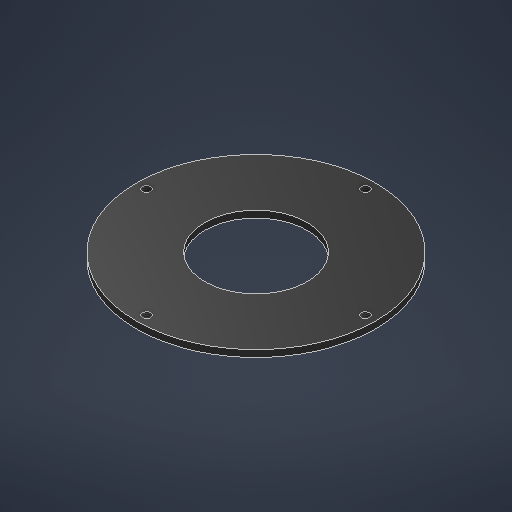
# Autodesk Inventor part: STRAIN_WAVE_BASS_PLATE,REV-ENG
Saved by Autodesk Inventor 2026.2 (Build 302298010, 298A)
## iProperties
Created: 2026-03-06
Part Number: STRAIN_WAVE_BASS_PLATE,REV-ENG
Material: Steel, 4140
Document SubType Name: Sheet Metal
Designer: 4aida
Density: 7.87 g/cm^3
Sheet Metal Rule: Default_mm
Appearance: Anodized - Dark Gray
Author: 4aida
Autodesk Inventor part; units mm, degrees
(part 1 of 3)
ref_plane "YZ Plane" through (0, 0, 0) normal (1, 0, 0) x (0, 1, 0)
ref_plane "XZ Plane" through (0, 0, 0) normal (0, 1, 0) x (-1, 0, 0)
ref_plane "XY Plane" through (0, 0, 0) normal (0, 0, 1) x (1, 0, 0)
sketch "Sketch1" plane through (0, 0, 0) normal (0, 1, 0) x (-1, 0, 0)
  circle A0 centre (0, 0) radius 15
  circle A1 centre (0, 0) radius 35
  dimension "d0" = 30
  dimension "d1" = 70
  measures "d0" diameter of A0
  measures "d1" diameter of A1
extrude "Plate1" add sketch "Sketch1" along normal blind 2
sketch "Sketch2" plane through (0, 0, 0) normal (0, -1, 0) x (1, 0, 0)
  line L0 (-32, -32) -> (32, -32)
  line L1 (32, -32) -> (32, 32)
  line L2 (32, 32) -> (-32, 32)
  line L3 (-32, 32) -> (-32, -32)
  line L4 (-32, -32) -> (32, 32) construction
  line L5 (32, -32) -> (-32, 32) construction
  point P0 (0, 0)
  point P1 (0, 32)
  point P2 (32, 0)
  point P3 (0, -32)
  point P4 (-32, 0)
  point P5 (32, 0)
  point P6 (0, -32)
  point P7 (-32, 0)
  point P8 (0, 32)
  dimension "d3" = 64
  constraints: 12 end point, 6 midpoint, 4 coincident, 2 parallel, 2 perpendicular, 1 horizontal
  measures "d3" distance between parallel lines of L3 L1
hole "Hole1" at (0, 0, 32) at (32, 0, 0) at (0, 0, -32) at (-32, 0, 0) direction (0, 1, 0) diameter 2.459 end through all thread size "M3x0.5" class "6H" standard "ANSI Metric M Profile"
sketch "Sketch3" plane through (0, 0, 0) normal (0, -1, 0) x (1, 0, 0)
  circle A0 centre (0, 0) radius 24.2903
  spline S0 degree 2 poles (5.459, -24.9705) (5.3721, -24.6393) (5.5007, -24.0358) (5.6869, -23.8278) knots 0 0 0 1 2 2 2
  spline S1 degree 2 poles (5.6869, -23.8278) (5.8408, -23.6638) (6.1984, -23.4862) (6.4923, -23.409) knots 0 0 0 1 2 2 2
  line L0 (6.4923, -23.409) -> (7.0489, -23.263)
  line L1 (7.0489, -23.263) -> (7.6835, -25.6811)
  line L2 (7.6835, -25.6811) -> (7.1328, -25.8256)
  spline S2 degree 2 poles (7.1328, -25.8256) (6.7919, -25.9151) (6.3771, -25.915) (6.2163, -25.8609) knots 0 0 0 1 2 2 2
  spline S3 degree 2 poles (6.2163, -25.8609) (5.9425, -25.7673) (5.5516, -25.3232) (5.459, -24.9705) knots 0 0 0 1 2 2 2
  spline S4 degree 2 poles (5.7951, -24.8864) (5.8681, -25.1647) (6.1557, -25.5102) (6.3673, -25.5741) knots 0 0 0 1 2 2 2
  spline S5 degree 2 poles (6.3673, -25.5741) (6.5166, -25.6166) (6.8266, -25.6085) (7.0441, -25.5515) knots 0 0 0 1 2 2 2
  line L3 (7.0441, -25.5515) -> (7.2891, -25.4872)
  line L4 (7.2891, -25.4872) -> (6.8005, -23.6256)
  line L5 (6.8005, -23.6256) -> (6.5556, -23.6899)
  spline S6 degree 2 poles (6.5556, -23.6899) (6.342, -23.7459) (6.0366, -23.8994) (5.9295, -24.0259) knots 0 0 0 1 2 2 2
  spline S7 degree 2 poles (5.9295, -24.0259) (5.7908, -24.1838) (5.721, -24.6043) (5.7951, -24.8864) knots 0 0 0 1 2 2 2
  line L6 (4.7869, -23.8246) -> (5.2074, -26.289)
  line L7 (5.2074, -26.289) -> (3.6657, -26.5521)
  line L8 (3.6657, -26.5521) -> (3.6159, -26.2605)
  line L9 (3.6159, -26.2605) -> (4.8301, -26.0533)
  line L10 (4.8301, -26.0533) -> (4.7149, -25.3783)
  line L11 (4.7149, -25.3783) -> (3.5826, -25.5715)
  line L12 (3.5826, -25.5715) -> (3.5328, -25.2799)
  line L13 (3.5328, -25.2799) -> (4.6652, -25.0867)
  line L14 (4.6652, -25.0867) -> (4.5091, -24.172)
  line L15 (4.5091, -24.172) -> (3.2949, -24.3792)
  line L16 (3.2949, -24.3792) -> (3.2451, -24.0877)
  line L17 (3.2451, -24.0877) -> (4.7869, -23.8246)
  spline S8 degree 2 poles (2.1849, -24.1471) (2.4553, -24.1227) (2.8448, -24.2015) (3.0196, -24.2671) knots 0 0 0 1 2 2 2
  line L18 (3.0196, -24.2671) -> (3.0571, -24.6828)
  line L19 (3.0571, -24.6828) -> (3.0329, -24.6849)
  spline S9 degree 2 poles (3.0329, -24.6849) (2.8556, -24.5463) (2.4267, -24.4141) (2.235, -24.4314) knots 0 0 0 1 2 2 2
  spline S10 degree 2 poles (2.235, -24.4314) (1.9606, -24.4562) (1.7007, -24.7095) (1.7176, -24.8971) knots 0 0 0 1 2 2 2
  spline S11 degree 2 poles (1.7176, -24.8971) (1.7311, -25.0464) (1.8951, -25.2188) (2.0587, -25.2508) knots 0 0 0 1 2 2 2
  spline S12 degree 2 poles (2.0587, -25.2508) (2.1766, -25.2727) (2.3723, -25.2998) (2.5188, -25.3232) knots 0 0 0 1 2 2 2
  spline S13 degree 2 poles (2.5188, -25.3232) (2.6511, -25.3459) (2.8641, -25.4304) (2.9503, -25.506) knots 0 0 0 1 2 2 2
  spline S14 degree 2 poles (2.9503, -25.506) (3.0344, -25.5819) (3.1392, -25.7962) (3.1523, -25.9414) knots 0 0 0 1 2 2 2
  spline S15 degree 2 poles (3.1523, -25.9414) (3.1796, -26.2441) (2.7444, -26.6963) (2.3792, -26.7292) knots 0 0 0 1 2 2 2
  spline S16 degree 2 poles (2.3792, -26.7292) (2.1693, -26.7482) (1.7906, -26.6989) (1.6241, -26.6346) knots 0 0 0 1 2 2 2
  line L20 (1.6241, -26.6346) -> (1.5884, -26.2391)
  line L21 (1.5884, -26.2391) -> (1.6126, -26.2369)
  spline S17 degree 2 poles (1.6126, -26.2369) (1.7415, -26.3352) (2.1273, -26.4631) (2.3311, -26.4447) knots 0 0 0 1 2 2 2
  spline S18 degree 2 poles (2.3311, -26.4447) (2.5612, -26.424) (2.8262, -26.1824) (2.8104, -26.0069) knots 0 0 0 1 2 2 2
  spline S19 degree 2 poles (2.8104, -26.0069) (2.7962, -25.8495) (2.6118, -25.6769) (2.4506, -25.6488) knots 0 0 0 1 2 2 2
  spline S20 degree 2 poles (2.4506, -25.6488) (2.3431, -25.63) (2.0319, -25.5848) (1.9282, -25.5636) knots 0 0 0 1 2 2 2
  spline S21 degree 2 poles (1.9282, -25.5636) (1.6649, -25.5081) (1.3982, -25.2128) (1.3773, -24.9807) knots 0 0 0 1 2 2 2
  spline S22 degree 2 poles (1.3773, -24.9807) (1.364, -24.8334) (1.4576, -24.5402) (1.5556, -24.4317) knots 0 0 0 1 2 2 2
  spline S23 degree 2 poles (1.5556, -24.4317) (1.6648, -24.312) (1.9569, -24.1677) (2.1849, -24.1471) knots 0 0 0 1 2 2 2
  line L22 (0.1039, -24.2949) -> (1.072, -24.2715)
  line L23 (1.072, -24.2715) -> (1.0782, -24.5267)
  line L24 (1.0782, -24.5267) -> (0.7602, -24.5344)
  line L25 (0.7602, -24.5344) -> (0.8083, -26.5233)
  line L26 (0.8083, -26.5233) -> (1.1263, -26.5156)
  line L27 (1.1263, -26.5156) -> (1.1324, -26.7708)
  line L28 (1.1324, -26.7708) -> (0.1643, -26.7942)
  line L29 (0.1643, -26.7942) -> (0.1581, -26.539)
  line L30 (0.1581, -26.539) -> (0.4761, -26.5313)
  line L31 (0.4761, -26.5313) -> (0.4281, -24.5424)
  line L32 (0.4281, -24.5424) -> (0.1101, -24.5501)
  line L33 (0.1101, -24.5501) -> (0.1039, -24.2949)
  spline S24 degree 2 poles (-1.3508, -24.2045) (-1.0857, -24.2176) (-0.6546, -24.4012) (-0.5049, -24.5729) knots 0 0 0 1 2 2 2
  spline S25 degree 2 poles (-0.5049, -24.5729) (-0.3553, -24.7467) (-0.2116, -25.2447) (-0.2273, -25.5623) knots 0 0 0 1 2 2 2
  spline S26 degree 2 poles (-0.2273, -25.5623) (-0.2422, -25.8638) (-0.4358, -26.333) (-0.602, -26.4951) knots 0 0 0 1 2 2 2
  spline S27 degree 2 poles (-0.602, -26.4951) (-0.7619, -26.6515) (-1.2159, -26.8076) (-1.4809, -26.7944) knots 0 0 0 1 2 2 2
  spline S28 degree 2 poles (-1.4809, -26.7944) (-1.6084, -26.7881) (-1.8373, -26.7403) (-1.9409, -26.7027) knots 0 0 0 1 2 2 2
  spline S29 degree 2 poles (-1.9409, -26.7027) (-2.0247, -26.6742) (-2.2267, -26.575) (-2.2878, -26.5395) knots 0 0 0 1 2 2 2
  line L34 (-2.2878, -26.5395) -> (-2.268, -26.1389)
  line L35 (-2.268, -26.1389) -> (-2.2397, -26.1403)
  spline S30 degree 2 poles (-2.2397, -26.1403) (-2.1796, -26.198) (-2.053, -26.3037) (-1.9344, -26.3663) knots 0 0 0 1 2 2 2
  spline S31 degree 2 poles (-1.9344, -26.3663) (-1.8357, -26.4219) (-1.578, -26.5016) (-1.4283, -26.509) knots 0 0 0 1 2 2 2
  spline S32 degree 2 poles (-1.4283, -26.509) (-1.0681, -26.5268) (-0.5961, -26.0066) (-0.5738, -25.5553) knots 0 0 0 1 2 2 2
  spline S33 degree 2 poles (-0.5738, -25.5553) (-0.5614, -25.3044) (-0.6601, -24.9223) (-0.765, -24.7873) knots 0 0 0 1 2 2 2
  spline S34 degree 2 poles (-0.765, -24.7873) (-0.8658, -24.6524) (-1.1626, -24.5019) (-1.3528, -24.4924) knots 0 0 0 1 2 2 2
  spline S35 degree 2 poles (-1.3528, -24.4924) (-1.4925, -24.4855) (-1.7737, -24.5122) (-1.8708, -24.548) knots 0 0 0 1 2 2 2
  line L36 (-1.8708, -24.548) -> (-1.9027, -25.1934)
  line L37 (-1.9027, -25.1934) -> (-1.324, -25.2221)
  line L38 (-1.324, -25.2221) -> (-1.3385, -25.5134)
  line L39 (-1.3385, -25.5134) -> (-2.245, -25.4686)
  line L40 (-2.245, -25.4686) -> (-2.191, -24.378)
  spline S36 degree 2 poles (-2.191, -24.378) (-2.1269, -24.3527) (-1.9081, -24.2763) (-1.8157, -24.2545) knots 0 0 0 1 2 2 2
  spline S37 degree 2 poles (-1.8157, -24.2545) (-1.6905, -24.2242) (-1.4904, -24.1976) (-1.3508, -24.2045) knots 0 0 0 1 2 2 2
  line L41 (-4.3677, -23.9111) -> (-3.9988, -23.9646)
  line L42 (-3.9988, -23.9646) -> (-3.2131, -26.2565)
  line L43 (-3.2131, -26.2565) -> (-2.9041, -24.1232)
  line L44 (-2.9041, -24.1232) -> (-2.5973, -24.1676)
  line L45 (-2.5973, -24.1676) -> (-2.9557, -26.6418)
  line L46 (-2.9557, -26.6418) -> (-3.4229, -26.5741)
  line L47 (-3.4229, -26.5741) -> (-4.1356, -24.4709)
  line L48 (-4.1356, -24.4709) -> (-4.4194, -26.4297)
  line L49 (-4.4194, -26.4297) -> (-4.7262, -26.3853)
  line L50 (-4.7262, -26.3853) -> (-4.3677, -23.9111)
  line L51 (-6.7505, -23.3385) -> (-5.815, -23.589)
  line L52 (-5.815, -23.589) -> (-5.8811, -23.8356)
  line L53 (-5.8811, -23.8356) -> (-6.1883, -23.7533)
  line L54 (-6.1883, -23.7533) -> (-6.703, -25.675)
  line L55 (-6.703, -25.675) -> (-6.3957, -25.7573)
  line L56 (-6.3957, -25.7573) -> (-6.4618, -26.0039)
  line L57 (-6.4618, -26.0039) -> (-7.3972, -25.7534)
  line L58 (-7.3972, -25.7534) -> (-7.3312, -25.5068)
  line L59 (-7.3312, -25.5068) -> (-7.0239, -25.5891)
  line L60 (-7.0239, -25.5891) -> (-6.5093, -23.6673)
  line L61 (-6.5093, -23.6673) -> (-6.8165, -23.585)
  line L62 (-6.8165, -23.585) -> (-6.7505, -23.3385)
  line L63 (-7.9724, -22.9498) -> (-7.0515, -23.2493)
  line L64 (-7.0515, -23.2493) -> (-7.1304, -23.4921)
  line L65 (-7.1304, -23.4921) -> (-7.4329, -23.3937)
  line L66 (-7.4329, -23.3937) -> (-8.0482, -25.2856)
  line L67 (-8.0482, -25.2856) -> (-7.7458, -25.384)
  line L68 (-7.7458, -25.384) -> (-7.8247, -25.6268)
  line L69 (-7.8247, -25.6268) -> (-8.7456, -25.3272)
  line L70 (-8.7456, -25.3272) -> (-8.6667, -25.0845)
  line L71 (-8.6667, -25.0845) -> (-8.3642, -25.1829)
  line L72 (-8.3642, -25.1829) -> (-7.7489, -23.2909)
  line L73 (-7.7489, -23.2909) -> (-8.0513, -23.1926)
  line L74 (-8.0513, -23.1926) -> (-7.9724, -22.9498)
  line L75 (-10.5093, -22.9446) -> (-9.6418, -23.3223)
  line L76 (-9.6418, -23.3223) -> (-9.7632, -23.6009)
  line L77 (-9.7632, -23.6009) -> (-10.6306, -23.2232)
  line L78 (-10.6306, -23.2232) -> (-10.5093, -22.9446)
  line L79 (-11.6735, -22.3747) -> (-10.8266, -22.7965)
  line L80 (-10.8266, -22.7965) -> (-10.962, -23.0685)
  line L81 (-10.962, -23.0685) -> (-11.8089, -22.6467)
  line L82 (-11.8089, -22.6467) -> (-11.6735, -22.3747)
  line L83 (-12.8069, -21.7458) -> (-11.9827, -22.2106)
  line L84 (-11.9827, -22.2106) -> (-12.132, -22.4753)
  line L85 (-12.132, -22.4753) -> (-12.9561, -22.0106)
  line L86 (-12.9561, -22.0106) -> (-12.8069, -21.7458)
  line L87 (-15.1638, -19.0088) -> (-14.8145, -19.2621)
  line L88 (-14.8145, -19.2621) -> (-14.7585, -20.5312)
  line L89 (-14.7585, -20.5312) -> (-14.4502, -20.7547)
  line L90 (-14.4502, -20.7547) -> (-13.8663, -19.9493)
  line L91 (-13.8663, -19.9493) -> (-13.5973, -20.1443)
  line L92 (-13.5973, -20.1443) -> (-15.0646, -22.1685)
  line L93 (-15.0646, -22.1685) -> (-15.5862, -21.7904)
  spline S38 degree 2 poles (-15.5862, -21.7904) (-15.7601, -21.6643) (-15.9673, -21.4566) (-16.024, -21.3104) knots 0 0 0 1 2 2 2
  spline S39 degree 2 poles (-16.024, -21.3104) (-16.0807, -21.1642) (-16.0479, -20.8602) (-15.9326, -20.701) knots 0 0 0 1 2 2 2
  spline S40 degree 2 poles (-15.9326, -20.701) (-15.7721, -20.4796) (-15.3281, -20.3435) (-15.0822, -20.4116) knots 0 0 0 1 2 2 2
  line L94 (-15.0822, -20.4116) -> (-15.1638, -19.0088)
  spline S41 degree 2 poles (-15.6366, -20.883) (-15.7008, -20.9716) (-15.7372, -21.1529) (-15.7037, -21.2448) knots 0 0 0 1 2 2 2
  spline S42 degree 2 poles (-15.7037, -21.2448) (-15.6736, -21.3241) (-15.5437, -21.4659) (-15.4321, -21.5467) knots 0 0 0 1 2 2 2
  line L95 (-15.4321, -21.5467) -> (-15.1648, -21.7405)
  line L96 (-15.1648, -21.7405) -> (-14.613, -20.9794)
  line L97 (-14.613, -20.9794) -> (-14.8493, -20.8082)
  spline S43 degree 2 poles (-14.8493, -20.8082) (-14.9657, -20.7238) (-15.1808, -20.6305) (-15.2911, -20.6481) knots 0 0 0 1 2 2 2
  spline S44 degree 2 poles (-15.2911, -20.6481) (-15.3906, -20.661) (-15.5605, -20.7781) (-15.6366, -20.883) knots 0 0 0 1 2 2 2
  line L98 (-15.3088, -18.8723) -> (-16.9399, -20.767)
  line L99 (-16.9399, -20.767) -> (-18.1252, -19.7466)
  line L100 (-18.1252, -19.7466) -> (-17.9322, -19.5224)
  line L101 (-17.9322, -19.5224) -> (-16.9987, -20.326)
  line L102 (-16.9987, -20.326) -> (-16.5519, -19.8071)
  line L103 (-16.5519, -19.8071) -> (-17.4225, -19.0576)
  line L104 (-17.4225, -19.0576) -> (-17.2295, -18.8335)
  line L105 (-17.2295, -18.8335) -> (-16.359, -19.5829)
  line L106 (-16.359, -19.5829) -> (-15.7536, -18.8797)
  line L107 (-15.7536, -18.8797) -> (-16.6871, -18.0761)
  line L108 (-16.6871, -18.0761) -> (-16.4941, -17.8519)
  line L109 (-16.4941, -17.8519) -> (-15.3088, -18.8723)
  line L110 (-19.812, -18.0627) -> (-17.4263, -16.9225)
  line L111 (-17.4263, -16.9225) -> (-17.1748, -17.178)
  line L112 (-17.1748, -17.178) -> (-18.3524, -19.5454)
  line L113 (-18.3524, -19.5454) -> (-18.6025, -19.2913)
  line L114 (-18.6025, -19.2913) -> (-17.6087, -17.3408)
  line L115 (-17.6087, -17.3408) -> (-19.5746, -18.3038)
  line L116 (-19.5746, -18.3038) -> (-19.812, -18.0627)
  line L117 (-18.2001, -16.1022) -> (-20.1202, -17.7032)
  line L118 (-20.1202, -17.7032) -> (-21.1218, -16.502)
  line L119 (-21.1218, -16.502) -> (-20.8947, -16.3126)
  line L120 (-20.8947, -16.3126) -> (-20.1058, -17.2586)
  line L121 (-20.1058, -17.2586) -> (-19.5799, -16.8201)
  line L122 (-19.5799, -16.8201) -> (-20.3156, -15.9378)
  line L123 (-20.3156, -15.9378) -> (-20.0884, -15.7484)
  line L124 (-20.0884, -15.7484) -> (-19.3527, -16.6306)
  line L125 (-19.3527, -16.6306) -> (-18.6401, -16.0364)
  line L126 (-18.6401, -16.0364) -> (-19.4289, -15.0904)
  line L127 (-19.4289, -15.0904) -> (-19.2018, -14.901)
  line L128 (-19.2018, -14.901) -> (-18.2001, -16.1022)
  line L129 (-20.5326, -13.0265) -> (-20.2849, -13.3798)
  line L130 (-20.2849, -13.3798) -> (-20.6458, -14.5978)
  line L131 (-20.6458, -14.5978) -> (-20.4271, -14.9096)
  line L132 (-20.4271, -14.9096) -> (-19.6126, -14.3386)
  line L133 (-19.6126, -14.3386) -> (-19.4219, -14.6106)
  line L134 (-19.4219, -14.6106) -> (-21.4689, -16.0458)
  line L135 (-21.4689, -16.0458) -> (-21.8388, -15.5183)
  spline S45 degree 2 poles (-21.8388, -15.5183) (-21.962, -15.3425) (-22.0902, -15.0785) (-22.0961, -14.9219) knots 0 0 0 1 2 2 2
  spline S46 degree 2 poles (-22.0961, -14.9219) (-22.1021, -14.7652) (-21.972, -14.4884) (-21.8111, -14.3756) knots 0 0 0 1 2 2 2
  spline S47 degree 2 poles (-21.8111, -14.3756) (-21.5871, -14.2186) (-21.1231, -14.2347) (-20.9128, -14.3792) knots 0 0 0 1 2 2 2
  line L136 (-20.9128, -14.3792) -> (-20.5326, -13.0265)
  spline S48 degree 2 poles (-21.5906, -14.6441) (-21.6802, -14.7069) (-21.7737, -14.8665) (-21.772, -14.9643) knots 0 0 0 1 2 2 2
  spline S49 degree 2 poles (-21.772, -14.9643) (-21.7694, -15.0491) (-21.6928, -15.2254) (-21.6137, -15.3382) knots 0 0 0 1 2 2 2
  line L137 (-21.6137, -15.3382) -> (-21.4241, -15.6086)
  line L138 (-21.4241, -15.6086) -> (-20.6544, -15.069)
  line L139 (-20.6544, -15.069) -> (-20.8219, -14.8301)
  spline S50 degree 2 poles (-20.8219, -14.8301) (-20.9044, -14.7123) (-21.0773, -14.554) (-21.1874, -14.5346) knots 0 0 0 1 2 2 2
  spline S51 degree 2 poles (-21.1874, -14.5346) (-21.2857, -14.5145) (-21.4845, -14.5697) (-21.5906, -14.6441) knots 0 0 0 1 2 2 2
  spline S52 degree 2 poles (-20.9377, -12.2257) (-20.8009, -12.4601) (-20.707, -12.8463) (-20.6922, -13.0324) knots 0 0 0 1 2 2 2
  line L140 (-20.6922, -13.0324) -> (-21.0527, -13.2427)
  line L141 (-21.0527, -13.2427) -> (-21.0649, -13.2217)
  spline S53 degree 2 poles (-21.0649, -13.2217) (-21.0146, -13.0024) (-21.077, -12.5579) (-21.174, -12.3916) knots 0 0 0 1 2 2 2
  spline S54 degree 2 poles (-21.174, -12.3916) (-21.3128, -12.1537) (-21.6525, -12.0258) (-21.8152, -12.1208) knots 0 0 0 1 2 2 2
  spline S55 degree 2 poles (-21.8152, -12.1208) (-21.9447, -12.1963) (-22.0312, -12.418) (-21.9907, -12.5797) knots 0 0 0 1 2 2 2
  spline S56 degree 2 poles (-21.9907, -12.5797) (-21.9605, -12.6958) (-21.902, -12.8845) (-21.861, -13.0271) knots 0 0 0 1 2 2 2
  spline S57 degree 2 poles (-21.861, -13.0271) (-21.8254, -13.1565) (-21.8116, -13.3853) (-21.8435, -13.4954) knots 0 0 0 1 2 2 2
  spline S58 degree 2 poles (-21.8435, -13.4954) (-21.8764, -13.6037) (-22.026, -13.7895) (-22.152, -13.8631) knots 0 0 0 1 2 2 2
  spline S59 degree 2 poles (-22.152, -13.8631) (-22.4145, -14.0162) (-23.0086, -13.814) (-23.1934, -13.4973) knots 0 0 0 1 2 2 2
  spline S60 degree 2 poles (-23.1934, -13.4973) (-23.2996, -13.3153) (-23.4157, -12.9515) (-23.4282, -12.7734) knots 0 0 0 1 2 2 2
  line L142 (-23.4282, -12.7734) -> (-23.0852, -12.5733)
  line L143 (-23.0852, -12.5733) -> (-23.0729, -12.5943)
  spline S61 degree 2 poles (-23.0729, -12.5943) (-23.1072, -12.7527) (-23.0593, -13.1563) (-22.9562, -13.3331) knots 0 0 0 1 2 2 2
  spline S62 degree 2 poles (-22.9562, -13.3331) (-22.8398, -13.5326) (-22.5086, -13.67) (-22.3563, -13.5812) knots 0 0 0 1 2 2 2
  spline S63 degree 2 poles (-22.3563, -13.5812) (-22.2199, -13.5016) (-22.1419, -13.2614) (-22.1848, -13.1034) knots 0 0 0 1 2 2 2
  spline S64 degree 2 poles (-22.1848, -13.1034) (-22.2134, -12.9981) (-22.3045, -12.6972) (-22.3294, -12.5944) knots 0 0 0 1 2 2 2
  spline S65 degree 2 poles (-22.3294, -12.5944) (-22.3908, -12.3323) (-22.2365, -11.9655) (-22.0353, -11.8481) knots 0 0 0 1 2 2 2
  spline S66 degree 2 poles (-22.0353, -11.8481) (-21.9076, -11.7736) (-21.6024, -11.7339) (-21.4625, -11.7766) knots 0 0 0 1 2 2 2
  spline S67 degree 2 poles (-21.4625, -11.7766) (-21.3078, -11.8247) (-21.0531, -12.0279) (-20.9377, -12.2257) knots 0 0 0 1 2 2 2
  line L144 (-21.5725, -11.1872) -> (-23.8245, -12.2727)
  line L145 (-23.8245, -12.2727) -> (-24.5036, -10.8638)
  line L146 (-24.5036, -10.8638) -> (-24.2372, -10.7354)
  line L147 (-24.2372, -10.7354) -> (-23.7023, -11.845)
  line L148 (-23.7023, -11.845) -> (-23.0855, -11.5477)
  line L149 (-23.0855, -11.5477) -> (-23.5842, -10.5129)
  line L150 (-23.5842, -10.5129) -> (-23.3178, -10.3844)
  line L151 (-23.3178, -10.3844) -> (-22.819, -11.4192)
  line L152 (-22.819, -11.4192) -> (-21.9832, -11.0163)
  line L153 (-21.9832, -11.0163) -> (-22.518, -9.9067)
  line L154 (-22.518, -9.9067) -> (-22.2515, -9.7783)
  line L155 (-22.2515, -9.7783) -> (-21.5725, -11.1872)
  line L156 (-22.7868, -8.4433) -> (-25.1554, -9.2429)
  line L157 (-25.1554, -9.2429) -> (-25.6557, -7.7611)
  line L158 (-25.6557, -7.7611) -> (-25.3754, -7.6665)
  line L159 (-25.3754, -7.6665) -> (-24.9814, -8.8335)
  line L160 (-24.9814, -8.8335) -> (-24.3327, -8.6145)
  line L161 (-24.3327, -8.6145) -> (-24.7001, -7.5261)
  line L162 (-24.7001, -7.5261) -> (-24.4198, -7.4315)
  line L163 (-24.4198, -7.4315) -> (-24.0524, -8.5199)
  line L164 (-24.0524, -8.5199) -> (-23.1733, -8.2231)
  line L165 (-23.1733, -8.2231) -> (-23.5673, -7.056)
  line L166 (-23.5673, -7.056) -> (-23.287, -6.9614)
  line L167 (-23.287, -6.9614) -> (-22.7868, -8.4433)
  line L168 (-23.8131, -4.8739) -> (-23.725, -5.2361)
  line L169 (-23.725, -5.2361) -> (-25.5579, -6.8205)
  line L170 (-25.5579, -6.8205) -> (-23.4635, -6.3109)
  line L171 (-23.4635, -6.3109) -> (-23.3902, -6.612)
  line L172 (-23.3902, -6.612) -> (-25.8193, -7.2031)
  line L173 (-25.8193, -7.2031) -> (-25.9309, -6.7444)
  line L174 (-25.9309, -6.7444) -> (-24.2457, -5.2981)
  line L175 (-24.2457, -5.2981) -> (-26.169, -5.7661)
  line L176 (-26.169, -5.7661) -> (-26.2422, -5.4649)
  line L177 (-26.2422, -5.4649) -> (-23.8131, -4.8739)
  spline S68 degree 2 poles (-24.0119, -3.3337) (-23.9737, -3.5963) (-24.0709, -4.0547) (-24.2106, -4.2346) knots 0 0 0 1 2 2 2
  spline S69 degree 2 poles (-24.2106, -4.2346) (-24.3523, -4.4149) (-24.8133, -4.6518) (-25.128, -4.6975) knots 0 0 0 1 2 2 2
  spline S70 degree 2 poles (-25.128, -4.6975) (-25.4268, -4.7409) (-25.9244, -4.6412) (-26.1155, -4.5093) knots 0 0 0 1 2 2 2
  spline S71 degree 2 poles (-26.1155, -4.5093) (-26.2998, -4.3825) (-26.5403, -3.9671) (-26.5784, -3.7045) knots 0 0 0 1 2 2 2
  spline S72 degree 2 poles (-26.5784, -3.7045) (-26.5968, -3.5782) (-26.5939, -3.3444) (-26.5769, -3.2354) knots 0 0 0 1 2 2 2
  spline S73 degree 2 poles (-26.5769, -3.2354) (-26.5651, -3.1477) (-26.5066, -2.9304) (-26.4836, -2.8636) knots 0 0 0 1 2 2 2
  line L178 (-26.4836, -2.8636) -> (-26.0866, -2.8059)
  line L179 (-26.0866, -2.8059) -> (-26.0825, -2.834)
  spline S74 degree 2 poles (-26.0825, -2.834) (-26.1276, -2.904) (-26.2069, -3.0486) (-26.2456, -3.1771) knots 0 0 0 1 2 2 2
  spline S75 degree 2 poles (-26.2456, -3.1771) (-26.2811, -3.2846) (-26.3097, -3.5528) (-26.2882, -3.7012) knots 0 0 0 1 2 2 2
  spline S76 degree 2 poles (-26.2882, -3.7012) (-26.2363, -4.0581) (-25.635, -4.4211) (-25.1879, -4.3561) knots 0 0 0 1 2 2 2
  spline S77 degree 2 poles (-25.1879, -4.3561) (-24.9393, -4.32) (-24.5832, -4.1496) (-24.471, -4.0207) knots 0 0 0 1 2 2 2
  spline S78 degree 2 poles (-24.471, -4.0207) (-24.3581, -3.8958) (-24.2674, -3.5755) (-24.2948, -3.3871) knots 0 0 0 1 2 2 2
  spline S79 degree 2 poles (-24.2948, -3.3871) (-24.3149, -3.2487) (-24.3952, -2.9779) (-24.449, -2.8895) knots 0 0 0 1 2 2 2
  line L180 (-24.449, -2.8895) -> (-25.0885, -2.9824)
  line L181 (-25.0885, -2.9824) -> (-25.0052, -3.5558)
  line L182 (-25.0052, -3.5558) -> (-25.294, -3.5977)
  line L183 (-25.294, -3.5977) -> (-25.4244, -2.6995)
  line L184 (-25.4244, -2.6995) -> (-24.3438, -2.5425)
  spline S80 degree 2 poles (-24.3438, -2.5425) (-24.3067, -2.6006) (-24.1896, -2.8006) (-24.1504, -2.887) knots 0 0 0 1 2 2 2
  spline S81 degree 2 poles (-24.1504, -2.887) (-24.0966, -3.0041) (-24.032, -3.1953) (-24.0119, -3.3337) knots 0 0 0 1 2 2 2
  line L185 (-24.2638, -1.2329) -> (-24.1955, -2.1988)
  line L186 (-24.1955, -2.1988) -> (-24.4501, -2.2169)
  line L187 (-24.4501, -2.2169) -> (-24.4725, -1.8996)
  line L188 (-24.4725, -1.8996) -> (-26.457, -2.04)
  line L189 (-26.457, -2.04) -> (-26.4346, -2.3573)
  line L190 (-26.4346, -2.3573) -> (-26.6892, -2.3753)
  line L191 (-26.6892, -2.3753) -> (-26.7576, -1.4094)
  line L192 (-26.7576, -1.4094) -> (-26.503, -1.3913)
  line L193 (-26.503, -1.3913) -> (-26.4805, -1.7086)
  line L194 (-26.4805, -1.7086) -> (-24.496, -1.5682)
  line L195 (-24.496, -1.5682) -> (-24.5185, -1.2509)
  line L196 (-24.5185, -1.2509) -> (-24.2638, -1.2329)
  line L197 (-24.2876, 0.9661) -> (-24.2887, 0.5933)
  line L198 (-24.2887, 0.5933) -> (-26.4475, -0.5065)
  line L199 (-26.4475, -0.5065) -> (-24.2919, -0.5129)
  line L200 (-24.2919, -0.5129) -> (-24.2928, -0.8228)
  line L201 (-24.2928, -0.8228) -> (-26.7928, -0.8154)
  line L202 (-26.7928, -0.8154) -> (-26.7914, -0.3434)
  line L203 (-26.7914, -0.3434) -> (-24.8091, 0.6576)
  line L204 (-24.8091, 0.6576) -> (-26.7885, 0.6635)
  line L205 (-26.7885, 0.6635) -> (-26.7876, 0.9734)
  line L206 (-26.7876, 0.9734) -> (-24.2876, 0.9661)
  line L207 (-24.2562, 1.4711) -> (-26.7461, 1.6954)
  line L208 (-26.7461, 1.6954) -> (-26.6057, 3.2531)
  line L209 (-26.6057, 3.2531) -> (-26.3111, 3.2266)
  line L210 (-26.3111, 3.2266) -> (-26.4217, 1.9998)
  line L211 (-26.4217, 1.9998) -> (-25.7397, 1.9384)
  line L212 (-25.7397, 1.9384) -> (-25.6366, 3.0824)
  line L213 (-25.6366, 3.0824) -> (-25.342, 3.0559)
  line L214 (-25.342, 3.0559) -> (-25.4451, 1.9118)
  line L215 (-25.4451, 1.9118) -> (-24.5209, 1.8286)
  line L216 (-24.5209, 1.8286) -> (-24.4104, 3.0554)
  line L217 (-24.4104, 3.0554) -> (-24.1158, 3.0288)
  line L218 (-24.1158, 3.0288) -> (-24.2562, 1.4711)
  line L219 (-24.0632, 3.3894) -> (-26.5275, 3.8104)
  line L220 (-26.5275, 3.8104) -> (-26.2641, 5.3521)
  line L221 (-26.2641, 5.3521) -> (-25.9725, 5.3023)
  line L222 (-25.9725, 5.3023) -> (-26.18, 4.0881)
  line L223 (-26.18, 4.0881) -> (-25.505, 3.9728)
  line L224 (-25.505, 3.9728) -> (-25.3115, 5.1051)
  line L225 (-25.3115, 5.1051) -> (-25.02, 5.0553)
  line L226 (-25.02, 5.0553) -> (-25.2134, 3.923)
  line L227 (-25.2134, 3.923) -> (-24.2988, 3.7668)
  line L228 (-24.2988, 3.7668) -> (-24.0914, 4.9809)
  line L229 (-24.0914, 4.9809) -> (-23.7998, 4.9311)
  line L230 (-23.7998, 4.9311) -> (-24.0632, 3.3894)
  line L231 (-23.238, 7.1603) -> (-23.346, 6.7425)
  line L232 (-23.346, 6.7425) -> (-24.5067, 6.2263)
  line L233 (-24.5067, 6.2263) -> (-24.6019, 5.8575)
  line L234 (-24.6019, 5.8575) -> (-23.6388, 5.6087)
  line L235 (-23.6388, 5.6087) -> (-23.7219, 5.287)
  line L236 (-23.7219, 5.287) -> (-26.1425, 5.9123)
  line L237 (-26.1425, 5.9123) -> (-25.9813, 6.536)
  spline S82 degree 2 poles (-25.9813, 6.536) (-25.9276, 6.744) (-25.8101, 7.0128) (-25.6947, 7.119) knots 0 0 0 1 2 2 2
  spline S83 degree 2 poles (-25.6947, 7.119) (-25.5794, 7.2252) (-25.2845, 7.306) (-25.0942, 7.2568) knots 0 0 0 1 2 2 2
  spline S84 degree 2 poles (-25.0942, 7.2568) (-24.8294, 7.1884) (-24.5403, 6.825) (-24.5138, 6.5713) knots 0 0 0 1 2 2 2
  line L238 (-24.5138, 6.5713) -> (-23.238, 7.1603)
  spline S85 degree 2 poles (-25.1553, 6.9148) (-25.2613, 6.9422) (-25.4433, 6.9097) (-25.5165, 6.8449) knots 0 0 0 1 2 2 2
  spline S86 degree 2 poles (-25.5165, 6.8449) (-25.5794, 6.7879) (-25.6638, 6.6151) (-25.6982, 6.4817) knots 0 0 0 1 2 2 2
  line L239 (-25.6982, 6.4817) -> (-25.7808, 6.162)
  line L240 (-25.7808, 6.162) -> (-24.8707, 5.9269)
  line L241 (-24.8707, 5.9269) -> (-24.7977, 6.2094)
  spline S87 degree 2 poles (-24.7977, 6.2094) (-24.7617, 6.3487) (-24.7535, 6.583) (-24.8103, 6.6792) knots 0 0 0 1 2 2 2
  spline S88 degree 2 poles (-24.8103, 6.6792) (-24.8587, 6.7671) (-25.0298, 6.8824) (-25.1553, 6.9148) knots 0 0 0 1 2 2 2
  line L242 (-22.8805, 8.1692) -> (-23.1879, 7.2509)
  line L243 (-23.1879, 7.2509) -> (-23.43, 7.332)
  line L244 (-23.43, 7.332) -> (-23.329, 7.6336)
  line L245 (-23.329, 7.6336) -> (-25.2156, 8.2651)
  line L246 (-25.2156, 8.2651) -> (-25.3165, 7.9635)
  line L247 (-25.3165, 7.9635) -> (-25.5586, 8.0446)
  line L248 (-25.5586, 8.0446) -> (-25.2512, 8.9629)
  line L249 (-25.2512, 8.9629) -> (-25.0091, 8.8818)
  line L250 (-25.0091, 8.8818) -> (-25.1101, 8.5802)
  line L251 (-25.1101, 8.5802) -> (-23.2235, 7.9486)
  line L252 (-23.2235, 7.9486) -> (-23.1225, 8.2503)
  line L253 (-23.1225, 8.2503) -> (-22.8805, 8.1692)
  line L254 (-22.0589, 10.2091) -> (-22.2029, 9.8652)
  line L255 (-22.2029, 9.8652) -> (-24.6185, 9.6777)
  line L256 (-24.6185, 9.6777) -> (-22.6302, 8.8449)
  line L257 (-22.6302, 8.8449) -> (-22.75, 8.559)
  line L258 (-22.75, 8.559) -> (-25.0559, 9.5249)
  line L259 (-25.0559, 9.5249) -> (-24.8735, 9.9603)
  line L260 (-24.8735, 9.9603) -> (-22.6589, 10.1243)
  line L261 (-22.6589, 10.1243) -> (-24.4845, 10.889)
  line L262 (-24.4845, 10.889) -> (-24.3648, 11.1749)
  line L263 (-24.3648, 11.1749) -> (-22.0589, 10.2091)
  spline S89 degree 2 poles (-21.3048, 11.5666) (-21.43, 11.3326) (-21.7802, 11.0214) (-21.9995, 10.9594) knots 0 0 0 1 2 2 2
  spline S90 degree 2 poles (-21.9995, 10.9594) (-22.2205, 10.8984) (-22.7321, 10.9813) (-23.0126, 11.1313) knots 0 0 0 1 2 2 2
  spline S91 degree 2 poles (-23.0126, 11.1313) (-23.2788, 11.2737) (-23.6201, 11.6492) (-23.6957, 11.8688) knots 0 0 0 1 2 2 2
  spline S92 degree 2 poles (-23.6957, 11.8688) (-23.7687, 12.0802) (-23.7158, 12.5573) (-23.5906, 12.7913) knots 0 0 0 1 2 2 2
  spline S93 degree 2 poles (-23.5906, 12.7913) (-23.5304, 12.9039) (-23.3894, 13.0903) (-23.3111, 13.1679) knots 0 0 0 1 2 2 2
  spline S94 degree 2 poles (-23.3111, 13.1679) (-23.2495, 13.2315) (-23.0735, 13.3717) (-23.0153, 13.4118) knots 0 0 0 1 2 2 2
  line L264 (-23.0153, 13.4118) -> (-22.6615, 13.2226)
  line L265 (-22.6615, 13.2226) -> (-22.6749, 13.1976)
  spline S95 degree 2 poles (-22.6749, 13.1976) (-22.7528, 13.168) (-22.9024, 13.0987) (-23.0098, 13.0183) knots 0 0 0 1 2 2 2
  spline S96 degree 2 poles (-23.0098, 13.0183) (-23.1022, 12.9528) (-23.2844, 12.7539) (-23.3551, 12.6217) knots 0 0 0 1 2 2 2
  spline S97 degree 2 poles (-23.3551, 12.6217) (-23.5251, 12.3037) (-23.2565, 11.6546) (-22.8581, 11.4416) knots 0 0 0 1 2 2 2
  spline S98 degree 2 poles (-22.8581, 11.4416) (-22.6366, 11.3231) (-22.2489, 11.249) (-22.082, 11.2862) knots 0 0 0 1 2 2 2
  spline S99 degree 2 poles (-22.082, 11.2862) (-21.9171, 11.3197) (-21.6541, 11.5237) (-21.5642, 11.6916) knots 0 0 0 1 2 2 2
  spline S100 degree 2 poles (-21.5642, 11.6916) (-21.4983, 11.8149) (-21.4022, 12.0805) (-21.393, 12.1836) knots 0 0 0 1 2 2 2
  line L266 (-21.393, 12.1836) -> (-21.9629, 12.4883)
  line L267 (-21.9629, 12.4883) -> (-22.2362, 11.9774)
  line L268 (-22.2362, 11.9774) -> (-22.4934, 12.115)
  line L269 (-22.4934, 12.115) -> (-22.0654, 12.9153)
  line L270 (-22.0654, 12.9153) -> (-21.1025, 12.4004)
  spline S101 degree 2 poles (-21.1025, 12.4004) (-21.1071, 12.3316) (-21.1316, 12.1012) (-21.1513, 12.0084) knots 0 0 0 1 2 2 2
  spline S102 degree 2 poles (-21.1513, 12.0084) (-21.1774, 11.8822) (-21.2389, 11.6899) (-21.3048, 11.5666) knots 0 0 0 1 2 2 2
  spline S103 degree 2 poles (-20.6525, 15.8798) (-20.5207, 15.7854) (-20.3508, 15.5217) (-20.3286, 15.3787) knots 0 0 0 1 2 2 2
  spline S104 degree 2 poles (-20.3286, 15.3787) (-20.3003, 15.1989) (-20.3973, 14.8373) (-20.553, 14.6199) knots 0 0 0 1 2 2 2
  line L271 (-20.553, 14.6199) -> (-20.717, 14.391)
  line L272 (-20.717, 14.391) -> (-19.9593, 13.8483)
  line L273 (-19.9593, 13.8483) -> (-20.1528, 13.5782)
  line L274 (-20.1528, 13.5782) -> (-22.1853, 15.0339)
  line L275 (-22.1853, 15.0339) -> (-21.8196, 15.5445)
  spline S105 degree 2 poles (-21.8196, 15.5445) (-21.6899, 15.7256) (-21.4489, 15.9368) (-21.3118, 15.9856) knots 0 0 0 1 2 2 2
  spline S106 degree 2 poles (-21.3118, 15.9856) (-21.153, 16.0438) (-20.8221, 16.0013) (-20.6525, 15.8798) knots 0 0 0 1 2 2 2
  spline S107 degree 2 poles (-20.846, 15.5922) (-20.9514, 15.6677) (-21.1581, 15.7061) (-21.2606, 15.6674) knots 0 0 0 1 2 2 2
  spline S108 degree 2 poles (-21.2606, 15.6674) (-21.3494, 15.6338) (-21.5067, 15.4873) (-21.5975, 15.3605) knots 0 0 0 1 2 2 2
  line L276 (-21.5975, 15.3605) -> (-21.7579, 15.1365)
  line L277 (-21.7579, 15.1365) -> (-20.9476, 14.5561)
  line L278 (-20.9476, 14.5561) -> (-20.8155, 14.7406)
  spline S109 degree 2 poles (-20.8155, 14.7406) (-20.6975, 14.9053) (-20.6051, 15.1456) (-20.6271, 15.2611) knots 0 0 0 1 2 2 2
  spline S110 degree 2 poles (-20.6271, 15.2611) (-20.6444, 15.3656) (-20.7488, 15.5226) (-20.846, 15.5922) knots 0 0 0 1 2 2 2
  line L279 (-17.7831, 16.5843) -> (-18.0625, 16.2555)
  line L280 (-18.0625, 16.2555) -> (-19.3322, 16.2976)
  line L281 (-19.3322, 16.2976) -> (-19.5788, 16.0073)
  line L282 (-19.5788, 16.0073) -> (-18.8208, 15.3632)
  line L283 (-18.8208, 15.3632) -> (-19.036, 15.11)
  line L284 (-19.036, 15.11) -> (-20.941, 16.7289)
  line L285 (-20.941, 16.7289) -> (-20.5238, 17.2199)
  spline S111 degree 2 poles (-20.5238, 17.2199) (-20.3847, 17.3835) (-20.1616, 17.5741) (-20.0115, 17.6193) knots 0 0 0 1 2 2 2
  spline S112 degree 2 poles (-20.0115, 17.6193) (-19.8614, 17.6646) (-19.5608, 17.6085) (-19.411, 17.4812) knots 0 0 0 1 2 2 2
  spline S113 degree 2 poles (-19.411, 17.4812) (-19.2026, 17.3041) (-19.1011, 16.851) (-19.188, 16.6111) knots 0 0 0 1 2 2 2
  line L286 (-19.188, 16.6111) -> (-17.7831, 16.5843)
  spline S114 degree 2 poles (-19.6153, 17.2002) (-19.6987, 17.271) (-19.8766, 17.3213) (-19.9708, 17.2949) knots 0 0 0 1 2 2 2
  spline S115 degree 2 poles (-19.9708, 17.2949) (-20.0522, 17.2711) (-20.2036, 17.1524) (-20.2928, 17.0475) knots 0 0 0 1 2 2 2
  line L287 (-20.2928, 17.0475) -> (-20.5066, 16.7958)
  line L288 (-20.5066, 16.7958) -> (-19.7903, 16.1871)
  line L289 (-19.7903, 16.1871) -> (-19.6014, 16.4094)
  spline S116 degree 2 poles (-19.6014, 16.4094) (-19.5083, 16.519) (-19.3986, 16.7262) (-19.4076, 16.8376) knots 0 0 0 1 2 2 2
  spline S117 degree 2 poles (-19.4076, 16.8376) (-19.4129, 16.9378) (-19.5165, 17.1162) (-19.6153, 17.2002) knots 0 0 0 1 2 2 2
  spline S118 degree 2 poles (-17.921, 19.5444) (-17.7035, 19.5244) (-17.251, 19.2864) (-17.0333, 19.063) knots 0 0 0 1 2 2 2
  spline S119 degree 2 poles (-17.0333, 19.063) (-16.8212, 18.8453) (-16.5879, 18.3853) (-16.5764, 18.1645) knots 0 0 0 1 2 2 2
  spline S120 degree 2 poles (-16.5764, 18.1645) (-16.5651, 17.9323) (-16.7408, 17.5291) (-16.9163, 17.358) knots 0 0 0 1 2 2 2
  spline S121 degree 2 poles (-16.9163, 17.358) (-17.0977, 17.1813) (-17.5081, 17.0218) (-17.7314, 17.039) knots 0 0 0 1 2 2 2
  spline S122 degree 2 poles (-17.7314, 17.039) (-17.9503, 17.0576) (-18.4013, 17.2999) (-18.6162, 17.5204) knots 0 0 0 1 2 2 2
  spline S123 degree 2 poles (-18.6162, 17.5204) (-18.8354, 17.7453) (-19.0574, 18.1966) (-19.0745, 18.4203) knots 0 0 0 1 2 2 2
  spline S124 degree 2 poles (-19.0745, 18.4203) (-19.086, 18.6411) (-18.9145, 19.0486) (-18.7346, 19.2239) knots 0 0 0 1 2 2 2
  spline S125 degree 2 poles (-18.7346, 19.2239) (-18.5518, 19.4021) (-18.1343, 19.56) (-17.921, 19.5444) knots 0 0 0 1 2 2 2
  spline S126 degree 2 poles (-17.2814, 18.8212) (-17.4539, 18.9982) (-17.798, 19.1975) (-17.9553, 19.2196) knots 0 0 0 1 2 2 2
  spline S127 degree 2 poles (-17.9553, 19.2196) (-18.1169, 19.2432) (-18.4076, 19.1409) (-18.5324, 19.0193) knots 0 0 0 1 2 2 2
  spline S128 degree 2 poles (-18.5324, 19.0193) (-18.6615, 18.8935) (-18.7683, 18.6141) (-18.749, 18.4462) knots 0 0 0 1 2 2 2
  spline S129 degree 2 poles (-18.749, 18.4462) (-18.731, 18.2855) (-18.5378, 17.9363) (-18.3681, 17.7622) knots 0 0 0 1 2 2 2
  spline S130 degree 2 poles (-18.3681, 17.7622) (-18.0246, 17.4096) (-17.3638, 17.3237) (-17.1157, 17.5655) knots 0 0 0 1 2 2 2
  spline S131 degree 2 poles (-17.1157, 17.5655) (-16.8675, 17.8072) (-16.9378, 18.4686) (-17.2814, 18.8212) knots 0 0 0 1 2 2 2
  spline S132 degree 2 poles (-15.5637, 19.4945) (-15.3541, 19.242) (-15.4349, 18.7114) (-15.6952, 18.4953) knots 0 0 0 1 2 2 2
  spline S133 degree 2 poles (-15.6952, 18.4953) (-15.7576, 18.4435) (-15.983, 18.2932) (-16.0661, 18.2506) knots 0 0 0 1 2 2 2
  line L290 (-16.0661, 18.2506) -> (-16.2706, 18.4968)
  line L291 (-16.2706, 18.4968) -> (-16.2565, 18.5085)
  spline S134 degree 2 poles (-16.2565, 18.5085) (-16.188, 18.5338) (-15.9943, 18.6208) (-15.9133, 18.6881) knots 0 0 0 1 2 2 2
  spline S135 degree 2 poles (-15.9133, 18.6881) (-15.7948, 18.7865) (-15.6983, 18.9588) (-15.707, 19.0359) knots 0 0 0 1 2 2 2
  spline S136 degree 2 poles (-15.707, 19.0359) (-15.7138, 19.1171) (-15.8194, 19.2822) (-15.9009, 19.3804) knots 0 0 0 1 2 2 2
  line L292 (-15.9009, 19.3804) -> (-16.8314, 20.5011)
  line L293 (-16.8314, 20.5011) -> (-17.2382, 20.1633)
  line L294 (-17.2382, 20.1633) -> (-17.4078, 20.3675)
  line L295 (-17.4078, 20.3675) -> (-16.7453, 20.9176)
  line L296 (-16.7453, 20.9176) -> (-15.5637, 19.4945)
  line L297 (-14.7657, 19.3003) -> (-16.226, 21.3294)
  line L298 (-16.226, 21.3294) -> (-14.9565, 22.243)
  line L299 (-14.9565, 22.243) -> (-14.7837, 22.0029)
  line L300 (-14.7837, 22.0029) -> (-15.7835, 21.2834)
  line L301 (-15.7835, 21.2834) -> (-15.3835, 20.7276)
  line L302 (-15.3835, 20.7276) -> (-14.4512, 21.3986)
  line L303 (-14.4512, 21.3986) -> (-14.2784, 21.1585)
  line L304 (-14.2784, 21.1585) -> (-15.2108, 20.4875)
  line L305 (-15.2108, 20.4875) -> (-14.6688, 19.7344)
  line L306 (-14.6688, 19.7344) -> (-13.669, 20.4539)
  line L307 (-13.669, 20.4539) -> (-13.4962, 20.2138)
  line L308 (-13.4962, 20.2138) -> (-14.7657, 19.3003)
  spline S137 degree 2 poles (-12.3306, 20.877) (-12.5389, 20.7517) (-12.9759, 20.6803) (-13.189, 20.7436) knots 0 0 0 1 2 2 2
  spline S138 degree 2 poles (-13.189, 20.7436) (-13.401, 20.8052) (-13.7923, 21.1372) (-13.9552, 21.408) knots 0 0 0 1 2 2 2
  spline S139 degree 2 poles (-13.9552, 21.408) (-14.1171, 21.6771) (-14.2202, 22.1589) (-14.1788, 22.3848) knots 0 0 0 1 2 2 2
  spline S140 degree 2 poles (-14.1788, 22.3848) (-14.137, 22.6061) (-13.8772, 22.9682) (-13.6602, 23.0987) knots 0 0 0 1 2 2 2
  spline S141 degree 2 poles (-13.6602, 23.0987) (-13.5526, 23.1635) (-13.3446, 23.2461) (-13.2501, 23.2698) knots 0 0 0 1 2 2 2
  spline S142 degree 2 poles (-13.2501, 23.2698) (-13.1671, 23.289) (-12.9844, 23.3115) (-12.8902, 23.3161) knots 0 0 0 1 2 2 2
  line L309 (-12.8902, 23.3161) -> (-12.6834, 22.9724)
  line L310 (-12.6834, 22.9724) -> (-12.706, 22.9588)
  spline S143 degree 2 poles (-12.706, 22.9588) (-12.7651, 22.9706) (-12.9416, 22.9968) (-13.0549, 22.9924) knots 0 0 0 1 2 2 2
  spline S144 degree 2 poles (-13.0549, 22.9924) (-13.1636, 22.9885) (-13.3908, 22.9298) (-13.5157, 22.8546) knots 0 0 0 1 2 2 2
  spline S145 degree 2 poles (-13.5157, 22.8546) (-13.6529, 22.7721) (-13.8298, 22.512) (-13.857, 22.349) knots 0 0 0 1 2 2 2
  spline S146 degree 2 poles (-13.857, 22.349) (-13.8815, 22.1854) (-13.7827, 21.7932) (-13.6584, 21.5866) knots 0 0 0 1 2 2 2
  spline S147 degree 2 poles (-13.6584, 21.5866) (-13.5257, 21.3662) (-13.2287, 21.1122) (-13.0709, 21.0582) knots 0 0 0 1 2 2 2
  spline S148 degree 2 poles (-13.0709, 21.0582) (-12.9169, 21.0066) (-12.6109, 21.0442) (-12.4755, 21.1256) knots 0 0 0 1 2 2 2
  spline S149 degree 2 poles (-12.4755, 21.1256) (-12.3522, 21.1998) (-12.1787, 21.3869) (-12.1243, 21.4812) knots 0 0 0 1 2 2 2
  spline S150 degree 2 poles (-12.1243, 21.4812) (-12.0733, 21.5733) (-12.0134, 21.737) (-12.0003, 21.7898) knots 0 0 0 1 2 2 2
  line L311 (-12.0003, 21.7898) -> (-11.9794, 21.8024)
  line L312 (-11.9794, 21.8024) -> (-11.7747, 21.4621)
  spline S151 degree 2 poles (-11.7747, 21.4621) (-11.8261, 21.3863) (-11.9145, 21.2504) (-11.9863, 21.1693) knots 0 0 0 1 2 2 2
  spline S152 degree 2 poles (-11.9863, 21.1693) (-12.0613, 21.0817) (-12.2022, 20.9543) (-12.3306, 20.877) knots 0 0 0 1 2 2 2
  line L313 (-10.8873, 21.7144) -> (-11.8616, 23.6916)
  line L314 (-11.8616, 23.6916) -> (-12.6139, 23.3209)
  line L315 (-12.6139, 23.3209) -> (-12.7447, 23.5862)
  line L316 (-12.7447, 23.5862) -> (-10.9419, 24.4745)
  line L317 (-10.9419, 24.4745) -> (-10.8112, 24.2092)
  line L318 (-10.8112, 24.2092) -> (-11.5635, 23.8384)
  line L319 (-11.5635, 23.8384) -> (-10.5893, 21.8612)
  line L320 (-10.5893, 21.8612) -> (-10.8873, 21.7144)
  line L321 (-8.1258, 23.8929) -> (-9.0156, 23.5715)
  line L322 (-9.0156, 23.5715) -> (-9.1189, 23.8573)
  line L323 (-9.1189, 23.8573) -> (-8.229, 24.1787)
  line L324 (-8.229, 24.1787) -> (-8.1258, 23.8929)
  line L325 (-6.8883, 24.2786) -> (-7.7935, 24.0033)
  line L326 (-7.7935, 24.0033) -> (-7.8819, 24.294)
  line L327 (-7.8819, 24.294) -> (-6.9768, 24.5693)
  line L328 (-6.9768, 24.5693) -> (-6.8883, 24.2786)
  line L329 (-5.6327, 24.6002) -> (-6.5508, 24.3718)
  line L330 (-6.5508, 24.3718) -> (-6.6242, 24.6666)
  line L331 (-6.6242, 24.6666) -> (-5.7061, 24.8951)
  line L332 (-5.7061, 24.8951) -> (-5.6327, 24.6002)
  line L333 (-3.3793, 24.0547) -> (-3.6709, 26.2395)
  line L334 (-3.6709, 26.2395) -> (-4.5022, 26.1286)
  line L335 (-4.5022, 26.1286) -> (-4.5414, 26.4218)
  line L336 (-4.5414, 26.4218) -> (-2.5493, 26.6876)
  line L337 (-2.5493, 26.6876) -> (-2.5102, 26.3944)
  line L338 (-2.5102, 26.3944) -> (-3.3415, 26.2835)
  line L339 (-3.3415, 26.2835) -> (-3.05, 24.0986)
  line L340 (-3.05, 24.0986) -> (-3.3793, 24.0547)
  line L341 (-1.9636, 24.2213) -> (-2.0926, 26.7179)
  line L342 (-2.0926, 26.7179) -> (-0.5307, 26.7986)
  line L343 (-0.5307, 26.7986) -> (-0.5154, 26.5032)
  line L344 (-0.5154, 26.5032) -> (-1.7455, 26.4397)
  line L345 (-1.7455, 26.4397) -> (-1.7102, 25.7558)
  line L346 (-1.7102, 25.7558) -> (-0.563, 25.8151)
  line L347 (-0.563, 25.8151) -> (-0.5477, 25.5197)
  line L348 (-0.5477, 25.5197) -> (-1.6949, 25.4604)
  line L349 (-1.6949, 25.4604) -> (-1.647, 24.5338)
  line L350 (-1.647, 24.5338) -> (-0.4169, 24.5974)
  line L351 (-0.4169, 24.5974) -> (-0.4016, 24.302)
  line L352 (-0.4016, 24.302) -> (-1.9636, 24.2213)
  line L353 (-0.3066, 24.3117) -> (0.6136, 26.7842)
  line L354 (0.6136, 26.7842) -> (1.0227, 26.7715)
  line L355 (1.0227, 26.7715) -> (1.7872, 24.2464)
  line L356 (1.7872, 24.2464) -> (1.4369, 24.2573)
  line L357 (1.4369, 24.2573) -> (1.2318, 24.963)
  line L358 (1.2318, 24.963) -> (0.2781, 24.9927)
  line L359 (0.2781, 24.9927) -> (0.0295, 24.3012)
  line L360 (0.0295, 24.3012) -> (-0.3066, 24.3117)
  line L361 (1.1496, 25.2493) -> (0.7994, 26.4379)
  line L362 (0.7994, 26.4379) -> (0.3781, 25.2734)
  line L363 (0.3781, 25.2734) -> (1.1496, 25.2493)
  line L364 (4.1812, 23.9517) -> (3.8517, 23.9944)
  line L365 (3.8517, 23.9944) -> (4.1282, 26.1301)
  line L366 (4.1282, 26.1301) -> (3.2932, 24.7612)
  line L367 (3.2932, 24.7612) -> (3.0923, 24.7873)
  line L368 (3.0923, 24.7873) -> (2.6394, 26.3229)
  line L369 (2.6394, 26.3229) -> (2.3629, 24.1871)
  line L370 (2.3629, 24.1871) -> (2.0555, 24.2269)
  line L371 (2.0555, 24.2269) -> (2.3765, 26.7062)
  line L372 (2.3765, 26.7062) -> (2.8265, 26.648)
  line L373 (2.8265, 26.648) -> (3.2667, 25.1875)
  line L374 (3.2667, 25.1875) -> (4.0441, 26.4903)
  line L375 (4.0441, 26.4903) -> (4.5022, 26.431)
  line L376 (4.5022, 26.431) -> (4.1812, 23.9517)
  spline S153 degree 2 poles (7.3944, 24.001) (7.3438, 23.8153) (7.1349, 23.5341) (7.0026, 23.4568) knots 0 0 0 1 2 2 2
  spline S154 degree 2 poles (7.0026, 23.4568) (6.8647, 23.3747) (6.5635, 23.3329) (6.4013, 23.3771) knots 0 0 0 1 2 2 2
  spline S155 degree 2 poles (6.4013, 23.3771) (6.2391, 23.4213) (6.0011, 23.6037) (5.9293, 23.7409) knots 0 0 0 1 2 2 2
  spline S156 degree 2 poles (5.9293, 23.7409) (5.8399, 23.9059) (5.819, 24.3841) (5.9063, 24.7046) knots 0 0 0 1 2 2 2
  spline S157 degree 2 poles (5.9063, 24.7046) (5.9921, 25.0193) (6.259, 25.4904) (6.445, 25.6413) knots 0 0 0 1 2 2 2
  spline S158 degree 2 poles (6.445, 25.6413) (6.6261, 25.7894) (7.0964, 25.8817) (7.3681, 25.8077) knots 0 0 0 1 2 2 2
  spline S159 degree 2 poles (7.3681, 25.8077) (7.4482, 25.7858) (7.5847, 25.7319) (7.6327, 25.6999) knots 0 0 0 1 2 2 2
  line L377 (7.6327, 25.6999) -> (7.548, 25.3891)
  line L378 (7.548, 25.3891) -> (7.5343, 25.3928)
  spline S160 degree 2 poles (7.5343, 25.3928) (7.4957, 25.4285) (7.3427, 25.5143) (7.2489, 25.5399) knots 0 0 0 1 2 2 2
  spline S161 degree 2 poles (7.2489, 25.5399) (6.9479, 25.6219) (6.4677, 25.316) (6.3238, 24.9268) knots 0 0 0 1 2 2 2
  spline S162 degree 2 poles (6.3238, 24.9268) (6.461, 24.9756) (6.7273, 24.9975) (6.872, 24.9581) knots 0 0 0 1 2 2 2
  spline S163 degree 2 poles (6.872, 24.9581) (7.0127, 24.9197) (7.2084, 24.8055) (7.3003, 24.6881) knots 0 0 0 1 2 2 2
  spline S164 degree 2 poles (7.3003, 24.6881) (7.406, 24.5522) (7.4509, 24.2082) (7.3944, 24.001) knots 0 0 0 1 2 2 2
  spline S165 degree 2 poles (7.0623, 24.0768) (7.1028, 24.2253) (7.0795, 24.448) (7.0126, 24.5418) knots 0 0 0 1 2 2 2
  spline S166 degree 2 poles (7.0126, 24.5418) (6.962, 24.6102) (6.8107, 24.6871) (6.7267, 24.71) knots 0 0 0 1 2 2 2
  spline S167 degree 2 poles (6.7267, 24.71) (6.6133, 24.7409) (6.3816, 24.7305) (6.2604, 24.6942) knots 0 0 0 1 2 2 2
  spline S168 degree 2 poles (6.2604, 24.6942) (6.2489, 24.6596) (6.2269, 24.5942) (6.213, 24.5434) knots 0 0 0 1 2 2 2
  spline S169 degree 2 poles (6.213, 24.5434) (6.1449, 24.2932) (6.159, 23.9596) (6.2114, 23.8593) knots 0 0 0 1 2 2 2
  spline S170 degree 2 poles (6.2114, 23.8593) (6.2591, 23.7644) (6.3911, 23.6633) (6.4752, 23.6404) knots 0 0 0 1 2 2 2
  spline S171 degree 2 poles (6.4752, 23.6404) (6.6706, 23.5872) (6.9867, 23.7992) (7.0623, 24.0768) knots 0 0 0 1 2 2 2
  spline S172 degree 2 poles (14.5804, -13.7754) (14.7669, -13.5781) (15.111, -13.3793) (15.2854, -13.3128) knots 0 0 0 1 2 2 2
  line L379 (15.2854, -13.3128) -> (15.5886, -13.5995)
  line L380 (15.5886, -13.5995) -> (15.5719, -13.6171)
  spline S173 degree 2 poles (15.5719, -13.6171) (15.3473, -13.6306) (14.9383, -13.8155) (14.8061, -13.9553) knots 0 0 0 1 2 2 2
  spline S174 degree 2 poles (14.8061, -13.9553) (14.6168, -14.1555) (14.5897, -14.5174) (14.7266, -14.6469) knots 0 0 0 1 2 2 2
  spline S175 degree 2 poles (14.7266, -14.6469) (14.8355, -14.7499) (15.0726, -14.7705) (15.2164, -14.6862) knots 0 0 0 1 2 2 2
  spline S176 degree 2 poles (15.2164, -14.6862) (15.3193, -14.6245) (15.4839, -14.5153) (15.6092, -14.4358) knots 0 0 0 1 2 2 2
  spline S177 degree 2 poles (15.6092, -14.4358) (15.7233, -14.3653) (15.939, -14.2876) (16.0536, -14.2872) knots 0 0 0 1 2 2 2
  spline S178 degree 2 poles (16.0536, -14.2872) (16.1669, -14.2884) (16.3873, -14.3796) (16.4932, -14.4798) knots 0 0 0 1 2 2 2
  spline S179 degree 2 poles (16.4932, -14.4798) (16.7141, -14.6886) (16.6872, -15.3156) (16.4353, -15.5821) knots 0 0 0 1 2 2 2
  spline S180 degree 2 poles (16.4353, -15.5821) (16.2905, -15.7352) (15.9741, -15.949) (15.8067, -16.011) knots 0 0 0 1 2 2 2
  line L381 (15.8067, -16.011) -> (15.5182, -15.7382)
  line L382 (15.5182, -15.7382) -> (15.5349, -15.7206)
  spline S181 degree 2 poles (15.5349, -15.7206) (15.6965, -15.7089) (16.0704, -15.5493) (16.2109, -15.4007) knots 0 0 0 1 2 2 2
  spline S182 degree 2 poles (16.2109, -15.4007) (16.3696, -15.2328) (16.4083, -14.8763) (16.2803, -14.7552) knots 0 0 0 1 2 2 2
  spline S183 degree 2 poles (16.2803, -14.7552) (16.1654, -14.6467) (15.913, -14.6394) (15.7735, -14.725) knots 0 0 0 1 2 2 2
  spline S184 degree 2 poles (15.7735, -14.725) (15.6805, -14.7821) (15.4174, -14.9543) (15.3257, -15.007) knots 0 0 0 1 2 2 2
  spline S185 degree 2 poles (15.3257, -15.007) (15.0915, -15.1397) (14.6962, -15.0949) (14.5269, -14.9348) knots 0 0 0 1 2 2 2
  spline S186 degree 2 poles (14.5269, -14.9348) (14.4194, -14.8332) (14.2954, -14.5515) (14.2971, -14.4053) knots 0 0 0 1 2 2 2
  spline S187 degree 2 poles (14.2971, -14.4053) (14.2997, -14.2433) (14.4231, -13.9417) (14.5804, -13.7754) knots 0 0 0 1 2 2 2
  line L383 (13.3205, -15.0575) -> (14.7672, -16.7206)
  line L384 (14.7672, -16.7206) -> (15.4, -16.1701)
  line L385 (15.4, -16.1701) -> (15.5941, -16.3933)
  line L386 (15.5941, -16.3933) -> (14.0778, -17.7123)
  line L387 (14.0778, -17.7123) -> (13.8836, -17.4891)
  line L388 (13.8836, -17.4891) -> (14.5165, -16.9387)
  line L389 (14.5165, -16.9387) -> (13.0699, -15.2756)
  line L390 (13.0699, -15.2756) -> (13.3205, -15.0575)
  line L391 (10.6478, -17.0886) -> (11.0007, -16.8403)
  line L392 (11.0007, -16.8403) -> (12.2193, -17.1994)
  line L393 (12.2193, -17.1994) -> (12.5308, -16.9803)
  line L394 (12.5308, -16.9803) -> (11.9586, -16.1667)
  line L395 (11.9586, -16.1667) -> (12.2303, -15.9756)
  line L396 (12.2303, -15.9756) -> (13.6685, -18.0204)
  line L397 (13.6685, -18.0204) -> (13.1416, -18.3911)
  spline S188 degree 2 poles (13.1416, -18.3911) (12.9659, -18.5146) (12.7021, -18.6432) (12.5455, -18.6493) knots 0 0 0 1 2 2 2
  spline S189 degree 2 poles (12.5455, -18.6493) (12.3888, -18.6555) (12.1118, -18.5258) (11.9988, -18.3651) knots 0 0 0 1 2 2 2
  spline S190 degree 2 poles (11.9988, -18.3651) (11.8414, -18.1413) (11.8568, -17.6773) (12.0011, -17.4668) knots 0 0 0 1 2 2 2
  line L398 (12.0011, -17.4668) -> (10.6478, -17.0886)
  spline S191 degree 2 poles (12.267, -18.1442) (12.3299, -18.2337) (12.4896, -18.327) (12.5874, -18.3251) knots 0 0 0 1 2 2 2
  spline S192 degree 2 poles (12.5874, -18.3251) (12.6722, -18.3224) (12.8485, -18.2455) (12.9611, -18.1662) knots 0 0 0 1 2 2 2
  line L399 (12.9611, -18.1662) -> (13.2313, -17.9763)
  line L400 (13.2313, -17.9763) -> (12.6905, -17.2074)
  line L401 (12.6905, -17.2074) -> (12.4518, -17.3752)
  spline S193 degree 2 poles (12.4518, -17.3752) (12.3342, -17.4579) (12.1761, -17.6311) (12.1569, -17.7412) knots 0 0 0 1 2 2 2
  spline S194 degree 2 poles (12.1569, -17.7412) (12.1369, -17.8394) (12.1924, -18.0382) (12.267, -18.1442) knots 0 0 0 1 2 2 2
  line L402 (10.7061, -17.0484) -> (11.1856, -19.6427)
  line L403 (11.1856, -19.6427) -> (10.828, -19.8417)
  line L404 (10.828, -19.8417) -> (8.8757, -18.0672)
  line L405 (8.8757, -18.0672) -> (9.182, -17.8967)
  line L406 (9.182, -17.8967) -> (9.7202, -18.3971)
  line L407 (9.7202, -18.3971) -> (10.5539, -17.933)
  line L408 (10.5539, -17.933) -> (10.4123, -17.2119)
  line L409 (10.4123, -17.2119) -> (10.7061, -17.0484)
  line L410 (9.9378, -18.6006) -> (10.8483, -19.4409)
  line L411 (10.8483, -19.4409) -> (10.6122, -18.2252)
  line L412 (10.6122, -18.2252) -> (9.9378, -18.6006)
  line L413 (7.8292, -18.5223) -> (8.7119, -18.1239)
  line L414 (8.7119, -18.1239) -> (8.8169, -18.3566)
  line L415 (8.8169, -18.3566) -> (8.527, -18.4874)
  line L416 (8.527, -18.4874) -> (9.3454, -20.3008)
  line L417 (9.3454, -20.3008) -> (9.6353, -20.1699)
  line L418 (9.6353, -20.1699) -> (9.7403, -20.4026)
  line L419 (9.7403, -20.4026) -> (8.8576, -20.8009)
  line L420 (8.8576, -20.8009) -> (8.7526, -20.5683)
  line L421 (8.7526, -20.5683) -> (9.0425, -20.4374)
  line L422 (9.0425, -20.4374) -> (8.2241, -18.6241)
  line L423 (8.2241, -18.6241) -> (7.9342, -18.7549)
  line L424 (7.9342, -18.7549) -> (7.8292, -18.5223)
  line L425 (5.7652, -19.2795) -> (6.1172, -19.157)
  line L426 (6.1172, -19.157) -> (7.8707, -20.829)
  line L427 (7.8707, -20.829) -> (7.1619, -18.7932)
  line L428 (7.1619, -18.7932) -> (7.4546, -18.6913)
  line L429 (7.4546, -18.6913) -> (8.2766, -21.0523)
  line L430 (8.2766, -21.0523) -> (7.8308, -21.2075)
  line L431 (7.8308, -21.2075) -> (6.2291, -19.6693)
  line L432 (6.2291, -19.6693) -> (6.8799, -21.5386)
  line L433 (6.8799, -21.5386) -> (6.5872, -21.6405)